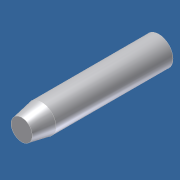
# Autodesk Inventor part: GE-12026-04
Saved by Autodesk Inventor 2012 (Build 160160000, 160)
## iProperties
Created: 2011-07-18
Part Number: GE-12026-04
Document SubType Name: Modeling
Designer: dfoster
Density: 1 g/cm^3
Description: Half Connector Pin
Material: Default
Title: Half Connector Pin
Author: dfoster
Autodesk Inventor part; units mm, degrees
ref_plane "YZ Plane" through (0, 0, 0) normal (1, 0, 0) x (0, 1, 0)
ref_plane "XZ Plane" through (0, 0, 0) normal (0, 1, 0) x (-1, 0, 0)
ref_plane "XY Plane" through (0, 0, 0) normal (0, 0, 1) x (1, 0, 0)
sketch "Sketch1" plane through (0, 0, 0) normal (0, 0, 1) x (1, 0, 0)
  circle A0 centre (0, 0) radius 18.2563
  dimension "d0" = 36.5125
  constraints: 1 centre point, 1 coincident
  measures "d0" diameter of A0
extrude "Extrusion1" add sketch "Sketch1" along normal blind 174.625
chamfer "Chamfer1" distance 25.4 distance2 4.7625 1 edges at (-18.2563, 0, 174.625) measured on face at (18.0198, -2.9285, 116.4167)
body "Solid1"
